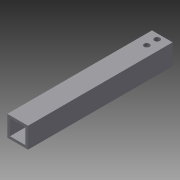
# Autodesk Inventor part: winch mount
Saved by Autodesk Inventor 2013 (Build 170138000, 138)
## iProperties
Created: 2013-02-03
Part Number: winch mount
Material: Aluminum 6061
Document SubType Name: Modeling
Designer: Arpan
Density: 1 g/cm^3
Mass: 49.7301 g
Surface Area: 321.601 cm^2
Volume: 49.7301 cm^3
Author: Arpan
Autodesk Inventor part; units mm, degrees
ref_plane "YZ Plane" through (0, 0, 0) normal (1, 0, 0) x (0, 1, 0)
ref_plane "XZ Plane" through (0, 0, 0) normal (0, 1, 0) x (-1, 0, 0)
ref_plane "XY Plane" through (0, 0, 0) normal (0, 0, 1) x (1, 0, 0)
sketch "Sketch1" plane through (0, 0, 0) normal (0, 0, 1) x (1, 0, 0)
  line L0 (0, 0) -> (-25.4, 0)
  line L1 (-25.4, 0) -> (-25.4, 25.4)
  line L2 (-25.4, 25.4) -> (0, 25.4)
  line L3 (0, 25.4) -> (0, 0)
  line L4 (-3.175, 22.225) -> (-22.225, 22.225)
  line L5 (-22.225, 22.225) -> (-22.225, 3.175)
  line L6 (-22.225, 3.175) -> (-3.175, 3.175)
  line L7 (-3.175, 3.175) -> (-3.175, 22.225)
  dimension "d0" = 25.4
  dimension "d2" = 25.4
  dimension "d3" = 3.175
  constraints: 16 end point, 4 parallel, 2 perpendicular, 1 horizontal, 3 other
  measures "d0" distance of L0.end L1.end
  measures "d2" distance of L0.start L0.end
  measures "d3" distance between parallel lines of L3 L7
extrude "Extrusion1" add sketch "Sketch1" along normal blind 177.8
sketch "Sketch2" plane through (-25.4, 25.4, 0) normal (0, 1, 0) x (1, 0, 0)
  circle A0 centre (12.7, -19.05) radius 3.3782 projected
  circle A1 centre (12.7, -6.35) radius 3.3782 projected
extrude "Extrusion2" cut sketch "Sketch2" against normal blind 25.4
body "Solid1"
